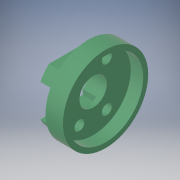
# Autodesk Inventor part: AS5047DEnclosureV2
Saved by Autodesk Inventor 2019.1 (Build 231200000, 200)
## iProperties
Created: 2018-06-30
Part Number: AS5047DEnclosureV2
Material: Generisch
Document SubType Name: Modeling
Designer: JochenAlt
Density: 1 g/cm^3
Appearance: Glatt - dunkelseegrün
Author: JochenAlt
Autodesk Inventor part; units mm, degrees
ref_plane "YZ Plane" through (0, 0, 0) normal (1, 0, 0) x (0, 1, 0)
ref_plane "XZ Plane" through (0, 0, 0) normal (0, 1, 0) x (-1, 0, 0)
ref_plane "XY Plane" through (0, 0, 0) normal (0, 0, 1) x (1, 0, 0)
ref_plane "Arbeitsebene1" through (0, 0, 0) normal (1, 0, 0) x (0, 0, -1)
sketch "Skizze1" plane through (0, 0, 0) normal (1, 0, 0) x (0, 0, -1)
  arc A0 (15.1, 0) -> (-15.1, 0) centre (0, 0) ccw
  circle A1 centre (0, 0) radius 5.5
  line L0 (-23.94, 0) -> (23.94, 0) construction
  line L1 (0, -23.94) -> (0, 23.94) construction
  line L2 (8.89, -5.5) -> (-8.89, -5.5) construction
  line L3 (-8.89, -5.5) -> (-8.89, 5.5) construction
  line L4 (-8.89, 5.5) -> (8.89, 5.5) construction
  line L5 (8.89, 5.5) -> (8.89, -5.5) construction
  circle A2 centre (8.89, 5.5) radius 1.2
  circle A3 centre (-8.89, 5.5) radius 1.2
  arc A4 (-15.1, 0) -> (14.6816, 3.5299) centre (0, 0) ccw
  line L6 (8.89, 7.7) -> (-8.89, 7.7)
  line L7 (6.5, 3.3) -> (6.5, 7.7)
  line L8 (-4.3414, 8.5633) -> (-4.3414, 8.4781)
  line L9 (-6.5, 7.7) -> (-6.5, 3.3)
  arc A5 (4.4, 3.3) -> (-4.4, 3.3) centre (0, 0) ccw
  line L10 (6.5, 3.3) -> (4.4, 3.3)
  line L11 (-4.4, 3.3) -> (-6.5, 3.3)
  line L12 (-6.5, -13.6294) -> (-6.5, -7.45)
  line L13 (6.5, -13.6294) -> (6.5, -7.45)
  line L14 (11.09, -10.248) -> (11.09, -7.45)
  circle A6 centre (8.89, -5.5) radius 1.2
  circle A7 centre (-8.89, -5.5) radius 1.2
  line L15 (11.09, -7.45) -> (11.09, 5.5)
  line L16 (-6.5, -7.45) -> (-6.5, 3.3)
  line L17 (-11.09, -7.45) -> (-11.09, 5.5)
  arc A8 (-8.89, 7.7) -> (-11.09, 5.5) centre (-8.89, 5.5) ccw
  arc A9 (11.09, 5.5) -> (8.89, 7.7) centre (8.89, 5.5) ccw
  arc A10 (7.7675, -7.45) -> (10.0125, -7.45) centre (8.89, -5.5) ccw
  line L18 (6.5, -7.45) -> (7.7675, -7.45)
  line L19 (10.0125, -7.45) -> (11.09, -7.45)
  arc A11 (-10.0125, -7.45) -> (-7.7675, -7.45) centre (-8.89, -5.5) ccw
  line L20 (-11.09, -7.45) -> (-10.0125, -7.45)
  line L21 (-7.7675, -7.45) -> (-6.5, -7.45)
  line L22 (6.5, -7.45) -> (6.5, 3.3)
  line L23 (-11.09, -7.45) -> (-11.09, -10.248)
  circle A12 centre (0, 0) radius 17.1
  circle A13 centre (-8.89, -5.5) radius 2
  circle A14 centre (8.89, -5.5) radius 2
  circle A15 centre (8.89, 5.5) radius 2
  circle A16 centre (-8.89, 5.5) radius 2
  point P0 (0, 15.1)
  dimension "d2" = 11
  dimension "d19" = 11
  dimension "d20" = 17.78
  dimension "d22" = 2.4
  dimension "d29" = 15.1
  dimension "d30" = 5.5
  dimension "d38" = 2.2
  dimension "d39" = 13
  dimension "d42" = 4.5
  dimension "d43" = 0.3
  dimension "d44" = 2
  dimension "d51" = 4
  constraints: 45 end point, 21 point on circle, 17 centre point, 17 coincident, 9 perpendicular, 8 equal radius, 7 collinear, 6 point on line, 4 tangent, 3 vertical, 2 parallel, 1 horizontal, 6 other
  measures "d2" diameter of A1
  measures "d19" distance of L2.end L3.end
  measures "d20" distance of L3.end L4.end
  measures "d22" diameter of A2
  measures "d29" radius of A4
  measures "d30" radius of A5
  measures "d38" radius of A8
  measures "d39" distance between parallel lines of L7 L9
  measures "d42" diameter of A10
  measures "d43" distance edge to line of A11 L20
  measures "d44" radial gap between concentric circles of A12 A4
  measures "d51" diameter of A13
extrude "Extrusion7" add sketch "Skizze1" along normal blind 2 contours A4 L14 L15 A9 L6 A8 L17 L23 A0 | A4 L13 L18 A10 L19 L14 | A4 L12 L16 L11 A1 L10 L22 L13 | L19 A10 L18 L22 L7 L6 A9 L15 | L23 L20 A11 L21 L12 A4 | L17 A8 L6 L9 L16 L21 A11 L20 | L10 A1 L11 L9 L6 L7 | A12
extrude "Extrusion3" add sketch "Skizze1" against normal blind 2.5 from surface at 0 contours A4 L13 L18 A10 L19 L14 | L19 A10 L18 L22 L7 L6 A9 L15 | L23 L20 A11 L21 L12 A4 | L17 A8 L6 L9 L16 L21 A11 L20 | L10 A1 L11 L9 L6 L7
extrude "Extrusion4" add sketch "Skizze1" against normal blind 3 from surface at -2.5 contours A4 L13 L18 A10 L19 L14 | L19 A10 L18 L22 L7 L6 A9 L15 | L23 L20 A11 L21 L12 A4 | L17 A8 L6 L9 L16 L21 A11 L20 | L10 A1 L11 L9 L6 L7 | A13 | A14 | A15 | A16
extrude "Extrusion8" add sketch "Skizze1" along normal blind 5 from surface at 2 contours A12
